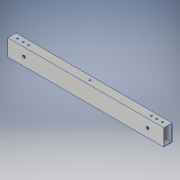
# Autodesk Inventor part: nhk18
Saved by Autodesk Inventor 2019 (Build 230136000, 136)
## iProperties
Created: 2022-02-15
Part Number: nhk18
Material: アルミニウム 6061
Document SubType Name: Sheet Metal
Designer: yuta
Density: 2.7 g/cm^3
Sheet Metal Rule: Default_mm
Appearance: アルミニウム - フラット
Author: yuta
Autodesk Inventor part; units mm, degrees
ref_plane "YZ Plane" through (0, 0, 0) normal (1, 0, 0) x (0, 1, 0)
ref_plane "XZ Plane" through (0, 0, 0) normal (0, 1, 0) x (-1, 0, 0)
ref_plane "XY Plane" through (0, 0, 0) normal (0, 0, 1) x (1, 0, 0)
sketch "スケッチ1" plane through (0, 0, 0) normal (1, 0, 0) x (0, 1, 0)
  line L0 (3.4879, 6.773) -> (-26.5121, 6.773)
  line L1 (-26.5121, 6.773) -> (-26.5121, -8.227)
  line L2 (-26.5121, -8.227) -> (3.4879, -8.227)
  line L3 (3.4879, -8.227) -> (3.4879, 6.773)
  point P0 (0, 0)
  dimension "d0" = 30
  dimension "d1" = 15
  constraints: 8 end point, 2 parallel, 1 horizontal, 1 perpendicular
  measures "d0" distance of L2.end L1.end
  measures "d1" distance of L1.end L0.end
extrude "押し出し1" add sketch "スケッチ1" along normal blind 280
sketch "スケッチ2" plane through (0, 3.4879, 6.773) normal (0, 1, 0) x (1, 0, 0)
  circle A0 centre (10, 7.5) radius 1.5
  line L0 (0, 15) -> (0, 0) projected
  line L1 (0, 15) -> (280, 15) projected
  circle A1 centre (20, 7.5) radius 1.5
  circle A2 centre (30, 7.5) radius 1.5
  circle A3 centre (270, 7.5) radius 1.5
  line L2 (280, 15) -> (280, 0) projected
  circle A4 centre (260, 7.5) radius 1.5
  circle A5 centre (250, 7.5) radius 1.5
  point P0 (0, 6.773)
  dimension "d4" = 3
  dimension "d5" = 10
  dimension "d6" = 7.5
  dimension "d7" = 3
  dimension "d8" = 3
  dimension "d9" = 10
  dimension "d10" = 10
  dimension "d11" = 3
  dimension "d12" = 10
  dimension "d13" = 3
  dimension "d14" = 3
  dimension "d15" = 10
  dimension "d16" = 10
  constraints: 6 centre point
  measures "d4" diameter of A0
  measures "d5" distance from line of L0 A0.centre
  measures "d6" distance from line of L1 A0.centre
  measures "d7" diameter of A1
  measures "d8" diameter of A2
  measures "d9" distance of A1.centre A0.centre
  measures "d10" distance of A2.centre A1.centre
  measures "d11" diameter of A3
  measures "d12" distance from line of L2 A3.centre
  measures "d13" diameter of A4
  measures "d14" diameter of A5
  measures "d15" distance of A3.centre A4.centre
  measures "d16" distance of A5.centre A4.centre
hole "穴1" at (270, 3.4879, -0.727) at (260, 3.4879, -0.727) at (250, 3.4879, -0.727) at (10, 3.4879, -0.727) at (20, 3.4879, -0.727) at (30, 3.4879, -0.727) direction (0, -1, 0) diameter 3 depth 30
sketch "スケッチ3" plane through (0, 0, 0) normal (-1, 0, 0) x (0, 0, 1)
  line L0 (-6.727, 1.9879) -> (5.273, 1.9879)
  line L1 (5.273, 1.9879) -> (5.273, -25.0121)
  line L2 (5.273, -25.0121) -> (-6.727, -25.0121)
  line L3 (-6.727, -25.0121) -> (-6.727, 1.9879)
  line L4 (-8.227, 3.4879) -> (6.773, 3.4879) projected
  line L5 (-8.227, -26.5121) -> (-8.227, 3.4879) projected
  point P0 (0, 0)
  dimension "d24" = 12
  dimension "d25" = 27
  dimension "d26" = 1.5
  dimension "d27" = 1.5
  constraints: 8 end point, 2 parallel, 1 horizontal, 1 perpendicular
  measures "d24" distance of L1.end L2.end
  measures "d25" distance of L0.end L1.end
  measures "d26" distance between parallel lines of L0 L4
  measures "d27" distance between parallel lines of L5 L3
extrude "押し出し2" cut sketch "スケッチ3" against normal blind 280
sketch "スケッチ4" plane through (0, 3.4879, 6.773) normal (0, 1, 0) x (1, 0, 0)
  circle A0 centre (140, 7.5) radius 1.5
  line L0 (0, 0) -> (280, 0) projected
  line L1 (0, 15) -> (0, 0) projected
  point P0 (0, 6.773)
  dimension "d30" = 3
  dimension "d31" = 7.5
  dimension "d32" = 140
  constraints: 1 centre point
  measures "d30" diameter of A0
  measures "d31" distance from line of L0 A0.centre
  measures "d32" distance from line of L1 A0.centre
hole "穴2" at (140, 3.4879, -0.727) direction (0, -1, 0) diameter 3 depth 30
sketch "スケッチ5" plane through (0, -26.5121, 6.773) normal (0, 0, 1) x (1, 0, 0)
  circle A0 centre (29, 15) radius 2.5
  line L0 (0, 30) -> (0, 0) projected
  line L1 (0, 30) -> (280, 30) projected
  point P0 (0, 26.5121)
  dimension "d40" = 5
  dimension "d41" = 29
  dimension "d42" = 15
  constraints: 1 centre point
  measures "d40" diameter of A0
  measures "d41" distance from line of L0 A0.centre
  measures "d42" distance from line of L1 A0.centre
hole "穴3" at (29, -11.5121, 6.773) direction (0, 0, -1) diameter 5 depth 15
sketch "スケッチ6" plane through (0, -26.5121, 6.773) normal (0, 0, 1) x (1, 0, 0)
  circle A0 centre (251, 15) radius 2.5
  line L0 (280, 30) -> (280, 0) projected
  line L1 (0, 30) -> (280, 30) projected
  point P0 (0, 26.5121)
  dimension "d50" = 5
  dimension "d51" = 29
  dimension "d52" = 15
  constraints: 1 centre point
  measures "d50" diameter of A0
  measures "d51" distance from line of L0 A0.centre
  measures "d52" distance from line of L1 A0.centre
hole "穴4" at (251, -11.5121, 6.773) direction (0, 0, -1) diameter 5 depth 15
equation "\"BendRadius\" = Thickness"
equation "\"BendReliefWidth\" = Thickness"
equation "\"BendReliefDepth\" = 0.5 * Thickness"
equation "\"CornerReliefSize\" = 4 * Thickness"
equation "\"MinimumRemnant\" = 2 * Thickness"
equation "\"TransitionRadius\" = BendRadius"
equation "\"JacobiRadiusSize\" = BendRadius"
equation "\"GapSize\" = Thickness"
equation "\"Thickness\" = 0.5"
